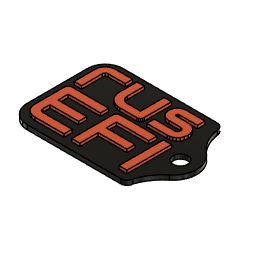
THIN - Keychain_v2 v1 (Autodesk Fusion 360 design; units mm, degrees)
Autodesk Fusion 360 part; units mm, degrees
note: some values were not read from the file. Set by a fixed rule: which sketch regions a step uses.
sketch "Sketch1" plane through (0, 0, 0) normal (0, 0, 1) x (1, 0, 0)
  line L0 (0, 0) -> (0, 17)
  line L1 (46.7294, 0) -> (46.7294, 50.0165)
  line L2 (9.2279, 24.9581) -> (3.5574, 24.9581)
  spline S0 degree 2 poles (3.5574, 24.9581) (3.0437, 24.9581) (2.7819, 24.7012) knots 0 0 0 1 1 1
  spline S1 degree 2 poles (2.7819, 24.7012) (2.5202, 24.4443) (2.5202, 23.95) knots 0 0 0 1 1 1
  line L3 (2.5202, 23.95) -> (2.5202, 17)
  line L4 (2.5202, 17) -> (0, 17)
  line L5 (0, 17) -> (0, 23.95)
  spline S2 degree 2 poles (0, 23.95) (0, 24.5994) (0.1648, 25.1132) knots 0 0 0 1 1 1
  spline S3 degree 2 poles (0.1648, 25.1132) (0.3296, 25.6269) (0.6058, 26.0195) knots 0 0 0 1 1 1
  spline S4 degree 2 poles (0.6058, 26.0195) (0.8821, 26.4121) (1.2407, 26.6883) knots 0 0 0 1 1 1
  spline S5 degree 2 poles (1.2407, 26.6883) (1.5994, 26.9646) (1.9919, 27.139) knots 0 0 0 1 1 1
  spline S6 degree 2 poles (1.9919, 27.139) (2.3845, 27.3135) (2.7868, 27.3959) knots 0 0 0 1 1 1
  spline S7 degree 2 poles (2.7868, 27.3959) (3.1891, 27.4783) (3.538, 27.4783) knots 0 0 0 1 1 1
  line L6 (3.538, 27.4783) -> (9.2279, 27.4783)
  line L7 (9.2279, 27.4783) -> (9.2279, 24.9581)
  spline S8 degree 2 poles (22.3427, 18.2698) (22.3427, 17.9984) (22.2458, 17.7658) knots 0 0 0 1 1 1
  spline S9 degree 2 poles (22.2458, 17.7658) (22.1489, 17.5331) (21.9793, 17.3635) knots 0 0 0 1 1 1
  spline S10 degree 2 poles (21.9793, 17.3635) (21.8096, 17.1939) (21.5818, 17.0969) knots 0 0 0 1 1 1
  spline S11 degree 2 poles (21.5818, 17.0969) (21.354, 17) (21.0923, 17) knots 0 0 0 1 1 1
  line L8 (21.0923, 17) -> (15.3927, 17)
  spline S12 degree 2 poles (15.3927, 17) (14.9275, 17) (14.3992, 17.1066) knots 0 0 0 1 1 1
  spline S13 degree 2 poles (14.3992, 17.1066) (13.8709, 17.2132) (13.3572, 17.4507) knots 0 0 0 1 1 1
  spline S14 degree 2 poles (13.3572, 17.4507) (12.8434, 17.6882) (12.3636, 18.0517) knots 0 0 0 1 1 1
  spline S15 degree 2 poles (12.3636, 18.0517) (11.8838, 18.4152) (11.5252, 18.9338) knots 0 0 0 1 1 1
  spline S16 degree 2 poles (11.5252, 18.9338) (11.1665, 19.4524) (10.9484, 20.1309) knots 0 0 0 1 1 1
  spline S17 degree 2 poles (10.9484, 20.1309) (10.7303, 20.8094) (10.7303, 21.6624) knots 0 0 0 1 1 1
  line L9 (10.7303, 21.6624) -> (10.7303, 27.4783)
  line L10 (10.7303, 27.4783) -> (13.2506, 27.4783)
  line L11 (13.2506, 27.4783) -> (13.2506, 21.6624)
  spline S18 degree 2 poles (13.2506, 21.6624) (13.2506, 21.1681) (13.4202, 20.7755) knots 0 0 0 1 1 1
  spline S19 degree 2 poles (13.4202, 20.7755) (13.5898, 20.3829) (13.8806, 20.1018) knots 0 0 0 1 1 1
  spline S20 degree 2 poles (13.8806, 20.1018) (14.1714, 19.8207) (14.564, 19.6705) knots 0 0 0 1 1 1
  spline S21 degree 2 poles (14.564, 19.6705) (14.9566, 19.5202) (15.4121, 19.5202) knots 0 0 0 1 1 1
  line L12 (15.4121, 19.5202) -> (19.8225, 19.5202)
  line L13 (19.8225, 19.5202) -> (19.8225, 27.4783)
  line L14 (19.8225, 27.4783) -> (22.3427, 27.4783)
  line L15 (22.3427, 27.4783) -> (22.3427, 18.2698)
  spline S22 degree 2 poles (34.8372, 20.538) (34.8372, 19.8886) (34.6725, 19.37) knots 0 0 0 1 1 1
  spline S23 degree 2 poles (34.6725, 19.37) (34.5077, 18.8514) (34.2363, 18.4588) knots 0 0 0 1 1 1
  spline S24 degree 2 poles (34.2363, 18.4588) (33.9649, 18.0662) (33.6062, 17.79) knots 0 0 0 1 1 1
  spline S25 degree 2 poles (33.6062, 17.79) (33.2476, 17.5137) (32.855, 17.3393) knots 0 0 0 1 1 1
  spline S26 degree 2 poles (32.855, 17.3393) (32.4624, 17.1648) (32.0601, 17.0824) knots 0 0 0 1 1 1
  spline S27 degree 2 poles (32.0601, 17.0824) (31.6579, 17) (31.2992, 17) knots 0 0 0 1 1 1
  line L16 (31.2992, 17) -> (24.4752, 17)
  line L17 (24.4752, 17) -> (24.4752, 19.5202)
  line L18 (24.4752, 19.5202) -> (31.2798, 19.5202)
  spline S28 degree 2 poles (31.2798, 19.5202) (31.7936, 19.5202) (32.0553, 19.7819) knots 0 0 0 1 1 1
  spline S29 degree 2 poles (32.0553, 19.7819) (32.317, 20.0437) (32.317, 20.538) knots 0 0 0 1 1 1
  spline S30 degree 2 poles (32.317, 20.538) (32.2685, 21.5461) (31.2992, 21.5461) knots 0 0 0 1 1 1
  line L19 (31.2992, 21.5461) -> (27.3929, 21.5461)
  spline S31 degree 2 poles (27.3929, 21.5461) (26.5593, 21.5461) (25.9777, 21.8369) knots 0 0 0 1 1 1
  spline S32 degree 2 poles (25.9777, 21.8369) (25.3961, 22.1277) (25.0326, 22.5639) knots 0 0 0 1 1 1
  spline S33 degree 2 poles (25.0326, 22.5639) (24.6691, 23.0001) (24.5092, 23.5041) knots 0 0 0 1 1 1
  spline S34 degree 2 poles (24.5092, 23.5041) (24.3492, 24.0082) (24.3492, 24.4443) knots 0 0 0 1 1 1
  spline S35 degree 2 poles (24.3492, 24.4443) (24.3492, 25.2877) (24.6497, 25.8644) knots 0 0 0 1 1 1
  spline S36 degree 2 poles (24.6497, 25.8644) (24.9502, 26.4411) (25.4058, 26.7998) knots 0 0 0 1 1 1
  spline S37 degree 2 poles (25.4058, 26.7998) (25.8614, 27.1584) (26.3945, 27.3184) knots 0 0 0 1 1 1
  spline S38 degree 2 poles (26.3945, 27.3184) (26.9276, 27.4783) (27.3929, 27.4783) knots 0 0 0 1 1 1
  line L20 (27.3929, 27.4783) -> (33.5868, 27.4783)
  line L21 (33.5868, 27.4783) -> (33.5868, 24.9581)
  line L22 (33.5868, 24.9581) -> (27.4123, 24.9581)
  spline S39 degree 2 poles (27.4123, 24.9581) (27.2184, 24.9581) (27.1069, 24.9145) knots 0 0 0 1 1 1
  spline S40 degree 2 poles (27.1069, 24.9145) (26.9955, 24.8708) (26.9422, 24.7981) knots 0 0 0 1 1 1
  spline S41 degree 2 poles (26.9422, 24.7981) (26.8888, 24.7255) (26.8791, 24.6431) knots 0 0 0 1 1 1
  spline S42 degree 2 poles (26.8791, 24.6431) (26.8695, 24.5607) (26.8695, 24.4831) knots 0 0 0 1 1 1
  spline S43 degree 2 poles (26.8695, 24.4831) (26.8791, 24.328) (26.9276, 24.2408) knots 0 0 0 1 1 1
  spline S44 degree 2 poles (26.9276, 24.2408) (26.9761, 24.1536) (27.0488, 24.1148) knots 0 0 0 1 1 1
  spline S45 degree 2 poles (27.0488, 24.1148) (27.1215, 24.076) (27.2136, 24.0712) knots 0 0 0 1 1 1
  spline S46 degree 2 poles (27.2136, 24.0712) (27.3056, 24.0663) (27.3929, 24.0663) knots 0 0 0 1 1 1
  line L23 (27.3929, 24.0663) -> (31.2992, 24.0663)
  spline S47 degree 2 poles (31.2992, 24.0663) (32.2685, 24.0663) (32.9471, 23.7174) knots 0 0 0 1 1 1
  spline S48 degree 2 poles (32.9471, 23.7174) (33.6256, 23.3684) (34.0424, 22.8401) knots 0 0 0 1 1 1
  spline S49 degree 2 poles (34.0424, 22.8401) (34.4592, 22.3119) (34.6482, 21.6915) knots 0 0 0 1 1 1
  spline S50 degree 2 poles (34.6482, 21.6915) (34.8372, 21.0711) (34.8372, 20.538) knots 0 0 0 1 1 1
  line L24 (12.3954, 6.1297) -> (2.7197, 6.1297)
  line L25 (2.7197, 8.8703) -> (12.3954, 8.8703)
  line L26 (12.3954, 8.8703) -> (12.3954, 6.1297)
  line L27 (13.6192, 0) -> (3.8075, 0)
  spline S51 degree 2 poles (3.8075, 0) (3.2427, 0) (2.5732, 0.1987) knots 0 0 0 1 1 1
  spline S52 degree 2 poles (2.5732, 0.1987) (1.9038, 0.3975) (1.3337, 0.8525) knots 0 0 0 1 1 1
  spline S53 degree 2 poles (1.3337, 0.8525) (0.7636, 1.3075) (0.3818, 2.0345) knots 0 0 0 1 1 1
  spline S54 degree 2 poles (0.3818, 2.0345) (0, 2.7615) (0, 3.818) knots 0 0 0 1 1 1
  line L28 (0, 3.818) -> (0, 13.6297)
  spline S55 degree 2 poles (0, 13.6297) (0, 13.9121) (0.1046, 14.1632) knots 0 0 0 1 1 1
  spline S56 degree 2 poles (0.1046, 14.1632) (0.2092, 14.4142) (0.3923, 14.6025) knots 0 0 0 1 1 1
  spline S57 degree 2 poles (0.3923, 14.6025) (0.5753, 14.7908) (0.8264, 14.8954) knots 0 0 0 1 1 1
  spline S58 degree 2 poles (0.8264, 14.8954) (1.0774, 15) (1.3703, 15) knots 0 0 0 1 1 1
  line L29 (1.3703, 15) -> (13.6192, 15)
  line L30 (13.6192, 15) -> (13.6192, 12.2803)
  line L31 (13.6192, 12.2803) -> (2.7197, 12.2803)
  spline S59 degree 2 poles (2.7197, 3.818) (2.7197, 3.2845) (3.0021, 3.0021) knots 0 0 0 1 1 1
  spline S60 degree 2 poles (3.0021, 3.0021) (3.2845, 2.7197) (3.8285, 2.7197) knots 0 0 0 1 1 1
  line L32 (3.8285, 2.7197) -> (13.6192, 2.7197)
  line L33 (13.6192, 2.7197) -> (13.6192, 0)
  line L34 (28.6506, 6.1297) -> (18.9644, 6.1297)
  line L35 (18.9644, 8.8703) -> (28.6506, 8.8703)
  line L36 (28.6506, 8.8703) -> (28.6506, 6.1297)
  line L37 (29.864, 12.2803) -> (18.9644, 12.2803)
  line L38 (18.9644, 0) -> (16.2448, 0)
  line L39 (16.2448, 0) -> (16.2448, 13.6297)
  spline S61 degree 2 poles (16.2448, 13.6297) (16.2448, 13.9121) (16.3494, 14.1632) knots 0 0 0 1 1 1
  spline S62 degree 2 poles (16.3494, 14.1632) (16.454, 14.4142) (16.637, 14.6025) knots 0 0 0 1 1 1
  spline S63 degree 2 poles (16.637, 14.6025) (16.8201, 14.7908) (17.0711, 14.8954) knots 0 0 0 1 1 1
  spline S64 degree 2 poles (17.0711, 14.8954) (17.3222, 15) (17.6151, 15) knots 0 0 0 1 1 1
  line L40 (17.6151, 15) -> (29.864, 15)
  line L41 (29.864, 15) -> (29.864, 12.2803)
  line L42 (34.8013, 0) -> (32.0816, 0)
  line L43 (32.0816, 0) -> (32.0816, 15)
  line L44 (32.0816, 15) -> (34.8013, 15)
  line L45 (34.8013, 15) -> (34.8013, 0)
  line L46 (2.7197, 12.2803) -> (2.7197, 8.8703)
  line L47 (2.7197, 6.1297) -> (2.7197, 3.818)
  line L48 (18.9644, 12.2803) -> (18.9644, 8.8703)
  line L49 (18.9644, 6.1297) -> (18.9644, 0)
  constraint coincident L24.end L46
  constraint coincident L34.end L48
  constraint collinear L46 L47
  constraint collinear L48 L49
sketch "Sketch2" plane through (0, 0, 0) normal (0, 0, 1) x (1, 0, 0)
  line L0 (3.538, 29.9783) -> (35.2726, 29.9781)
  line L1 (-2.5, 3.818) -> (-2.5, 23.95)
  spline S0 degree 3 poles (-2.5, 23.95) (-2.5, 24.5944) (-2.4192, 25.2425) (-2.2158, 25.8767) knots 0 0 0 0 1 1 1 1
  spline S1 degree 3 poles (-2.2158, 25.8767) (-2.0384, 26.4298) (-1.7836, 26.9681) (-1.4387, 27.4582) knots 0 0 0 0 1 1 1 1
  spline S2 degree 3 poles (-1.4387, 27.4582) (-1.1203, 27.9106) (-0.7316, 28.3247) (-0.2848, 28.6689) knots 0 0 0 0 1 1 1 1
  spline S3 degree 3 poles (-0.2848, 28.6689) (0.102, 28.9669) (0.5256, 29.2231) (0.9766, 29.4236) knots 0.000003 0.000003 0.000003 0.000003 1 1 1 1
  spline S4 degree 3 poles (0.9766, 29.4236) (1.3945, 29.6093) (1.8337, 29.7526) (2.2852, 29.8451) knots 0 0 0 0 1 1 1 1
  spline S5 degree 3 poles (2.2852, 29.8451) (2.6925, 29.9285) (3.1086, 29.9783) (3.538, 29.9783) knots 0.000006 0.000006 0.000006 0.000006 1 1 1 1
  line L2 (35.302, -2.5) -> (3.8075, -2.5)
  spline S6 degree 3 poles (3.8075, -2.5) (3.1378, -2.5) (2.4919, -2.385) (1.8617, -2.1979) knots 0 0 0 0 1 1 1 1
  spline S7 degree 3 poles (1.8617, -2.1979) (1.102, -1.9723) (0.3884, -1.5917) (-0.2259, -1.1014) knots 0.000003 0.000003 0.000003 0.000003 1 1 1 1
  spline S8 degree 3 poles (-0.2259, -1.1014) (-0.9006, -0.5629) (-1.4387, 0.1241) (-1.8315, 0.8721) knots 0.000002 0.000002 0.000002 0.000002 1 1 1 1
  spline S9 degree 3 poles (-1.8315, 0.8721) (-2.3179, 1.7981) (-2.5, 2.8125) (-2.5, 3.818) knots 0 0 0 0 1 1 1 1
  line L3 (37.3013, 12.981) -> (47.3013, 13.0001) construction
  circle A0 centre (41.3001, 12.886) radius 4 construction
  arc A1 (45.3013, 12.9963) -> (37.286, 20.981) centre (37.3013, 12.981) ccw
  line L4 (37.2726, 27.9819) -> (37.286, 20.981)
  line L5 (37.3013, 12.981) -> (37.3166, 4.981)
  line L6 (37.286, 20.981) -> (37.3013, 12.981)
  line L7 (37.3166, 4.981) -> (37.302, -0.5053)
  arc A2 (37.3166, 4.981) -> (45.3013, 12.9963) centre (37.3013, 12.981) ccw
  line L8 (37.2963, 15.5591) -> (37.2772, 25.5591) construction
  line L9 (37.3099, 8.4845) -> (37.329, -1.5154) construction
  arc A3 (35.302, -2.5) -> (37.302, -0.5053) centre (35.302, -0.5) ccw
  arc A4 (37.2726, 27.9819) -> (35.2726, 29.9781) centre (35.2726, 27.9781) ccw
  circle A5 centre (39.8013, 12.982) radius 2.5
  line L10 (42.3013, 12.9905) -> (42.2893, 19.2355) construction
  line L11 (42.3013, 12.9905) -> (42.3132, 6.7456) construction
  arc A6 (37.2726, 27.9819) -> (42.2893, 19.2355) centre (50.8322, 29.9474) ccw
  arc A7 (42.3132, 6.7456) -> (37.302, -0.5053) centre (52.0006, -5.3068) ccw
  dimension "d14" = 10
  dimension "d16" = 8
  dimension "d20" = 10
  dimension "d21" = 10
  dimension "d26" = 2
  dimension "d27" = 2
  dimension "d28" = 5
  constraint coincident S5 L0.start
  constraint coincident L0 S5.end
  constraint perpendicular L3 L4
  constraint coincident L3.start A0
  constraint coincident L3.start A1.centre
  constraint tangent A0 A1
  constraint coincident L5.end L4
  constraint coincident L3.start L4
  constraint coincident L3 A1.start
  constraint concentric A1 A2
  constraint coincident L6 L8.start
  constraint coincident L5 L9.start
  constraint tangent L2 A3
  constraint tangent L7 A3
  constraint tangent L0 A4
  constraint tangent L4 A4
  constraint coincident L3.start A5
  constraint midpoint L3 L10.start
  constraint coincident A1 L10.end
  constraint perpendicular L3 L10
  constraint coincident A2 L11.end
  constraint parallel L10 L11
  constraint tangent A1 A6
  constraint tangent A2 A7
  measures "d14" distance of L3.start L3.end
  measures "d16" diameter of A0
  measures "d20" distance of L8.start L8.end
  measures "d21" distance of L9.start L9.end
  measures "d26" radius of A3
  measures "d27" radius of A4
  measures "d28" diameter of A5
extrude "Extrude1" add sketch "Sketch1" along normal blind 2.5 makes body 1 at (17.1513, 6.5865, 0) makes body 2 at (1.6801, 19.3167, 0) makes body 3 at (33.8947, 5, 0) makes body 4 at (29.0181, 17.8401, 0) makes body 5 at (21.5027, 21.7561, 0) makes body 6 at (0.9066, 8.7727, 0)
extrude "Extrude2" cut sketch "Sketch2" along normal blind 1.5 contours L0 L1 S0 S1 S2 S3 S4 S5 L2 S6 S7 S8 S9 L4 L5 L6 L7 A3 A4 bodies 1 2 3 4 5 6
extrude "Extrude3" add sketch "Sketch2" along normal blind 1.5 separate body contours L0 L1 S0 S1 S2 S3 S4 S5 L2 S6 S7 S8 S9 L4 L5 L6 L7 A3 A4 makes body 7
extrude "Extrude5" add sketch "Sketch2" along normal up to surface (1.5 mm away) contours A1 L4 A6 | A1 L5 L6 A2 | L7 A2 A7 bodies 7
sketch "Sketch4" plane through (0, 0, 0) normal (0, 0, 1) x (1, 0, 0)
  line L0 (-2.5, 3.818) -> (-2.5, 23.95) construction
  line L1 (37.3013, 12.981) -> (-2.5, 12.981) construction
  spline S0 degree 2 poles (31.8619, 9.7118) (31.8619, 9.5612) (31.9205, 9.4301) knots 0 0 0 1 1 1
  spline S1 degree 2 poles (31.9205, 9.4301) (31.9791, 9.299) (32.0767, 9.2014) knots 0 0 0 1 1 1
  spline S2 degree 2 poles (32.0767, 9.2014) (32.1744, 9.1037) (32.3055, 9.0479) knots 0 0 0 1 1 1
  spline S3 degree 2 poles (32.3055, 9.0479) (32.4366, 8.9921) (32.5816, 8.9921) knots 0 0 0 1 1 1
  spline S4 degree 2 poles (32.5816, 8.9921) (32.7322, 8.9921) (32.8633, 9.0479) knots 0 0 0 1 1 1
  spline S5 degree 2 poles (32.8633, 9.0479) (32.9944, 9.1037) (33.0921, 9.2014) knots 0 0 0 1 1 1
  spline S6 degree 2 poles (33.0921, 9.2014) (33.1897, 9.299) (33.2455, 9.4301) knots 0 0 0 1 1 1
  spline S7 degree 2 poles (33.2455, 9.4301) (33.3013, 9.5612) (33.3013, 9.7118) knots 0 0 0 1 1 1
  spline S8 degree 2 poles (33.3013, 9.7118) (33.3013, 9.8569) (33.2455, 9.988) knots 0 0 0 1 1 1
  spline S9 degree 2 poles (33.2455, 9.988) (33.1897, 10.1191) (33.0921, 10.2167) knots 0 0 0 1 1 1
  spline S10 degree 2 poles (33.0921, 10.2167) (32.9944, 10.3143) (32.8633, 10.3729) knots 0 0 0 1 1 1
  spline S11 degree 2 poles (32.8633, 10.3729) (32.7322, 10.4315) (32.5816, 10.4315) knots 0 0 0 1 1 1
  spline S12 degree 2 poles (32.5816, 10.4315) (32.4366, 10.4315) (32.3055, 10.3729) knots 0 0 0 1 1 1
  spline S13 degree 2 poles (32.3055, 10.3729) (32.1744, 10.3143) (32.0767, 10.2167) knots 0 0 0 1 1 1
  spline S14 degree 2 poles (32.0767, 10.2167) (31.9791, 10.1191) (31.9205, 9.988) knots 0 0 0 1 1 1
  spline S15 degree 2 poles (31.9205, 9.988) (31.8619, 9.8569) (31.8619, 9.7118) knots 0 0 0 1 1 1
  line L2 (23.4045, 8.981) -> (28.6374, 8.981)
  spline S16 degree 2 poles (28.6374, 8.981) (28.8382, 8.981) (29.0698, 9.0284) knots 0 0 0 1 1 1
  spline S17 degree 2 poles (29.0698, 9.0284) (29.3013, 9.0758) (29.5272, 9.1762) knots 0 0 0 1 1 1
  spline S18 degree 2 poles (29.5272, 9.1762) (29.7532, 9.2767) (29.9596, 9.4357) knots 0 0 0 1 1 1
  spline S19 degree 2 poles (29.9596, 9.4357) (30.166, 9.5947) (30.325, 9.8206) knots 0 0 0 1 1 1
  spline S20 degree 2 poles (30.325, 9.8206) (30.484, 10.0465) (30.5788, 10.345) knots 0 0 0 1 1 1
  spline S21 degree 2 poles (30.5788, 10.345) (30.6737, 10.6435) (30.6737, 11.0173) knots 0 0 0 1 1 1
  line L3 (30.6737, 11.0173) -> (30.6737, 14.9447)
  spline S22 degree 2 poles (30.6737, 14.9447) (30.6737, 15.1456) (30.6262, 15.3771) knots 0 0 0 1 1 1
  spline S23 degree 2 poles (30.6262, 15.3771) (30.5788, 15.6086) (30.4784, 15.8345) knots 0 0 0 1 1 1
  spline S24 degree 2 poles (30.4784, 15.8345) (30.378, 16.0605) (30.2162, 16.2669) knots 0 0 0 1 1 1
  spline S25 degree 2 poles (30.2162, 16.2669) (30.0544, 16.4733) (29.8285, 16.6323) knots 0 0 0 1 1 1
  spline S26 degree 2 poles (29.8285, 16.6323) (29.6025, 16.7913) (29.3069, 16.8862) knots 0 0 0 1 1 1
  spline S27 degree 2 poles (29.3069, 16.8862) (29.0112, 16.981) (28.6374, 16.981) knots 0 0 0 1 1 1
  line L4 (28.6374, 16.981) -> (23.4045, 16.981)
  line L5 (23.4045, 16.981) -> (23.4045, 15.5305)
  line L6 (23.4045, 15.5305) -> (28.6374, 15.5305)
  spline S28 degree 2 poles (28.6374, 15.5305) (28.9219, 15.5305) (29.0725, 15.3799) knots 0 0 0 1 1 1
  spline S29 degree 2 poles (29.0725, 15.3799) (29.2232, 15.2292) (29.2232, 14.9336) knots 0 0 0 1 1 1
  line L7 (29.2232, 14.9336) -> (29.2232, 11.0173)
  spline S30 degree 2 poles (29.2232, 11.0173) (29.2232, 10.7383) (29.0698, 10.5849) knots 0 0 0 1 1 1
  spline S31 degree 2 poles (29.0698, 10.5849) (28.9163, 10.4315) (28.6374, 10.4315) knots 0 0 0 1 1 1
  line L8 (28.6374, 10.4315) -> (23.4045, 10.4315)
  line L9 (23.4045, 10.4315) -> (23.4045, 8.981)
  spline S32 degree 2 poles (13.636, 12.2167) (13.636, 11.4859) (13.887, 10.8722) knots 0 0 0 1 1 1
  spline S33 degree 2 poles (13.887, 10.8722) (14.1381, 10.2585) (14.5844, 9.8122) knots 0 0 0 1 1 1
  spline S34 degree 2 poles (14.5844, 9.8122) (15.0307, 9.3659) (15.6416, 9.1177) knots 0 0 0 1 1 1
  spline S35 degree 2 poles (15.6416, 9.1177) (16.2525, 8.8694) (16.9721, 8.8694) knots 0 0 0 1 1 1
  line L10 (16.9721, 8.8694) -> (18.9359, 8.8694)
  spline S36 degree 2 poles (18.9359, 8.8694) (19.6555, 8.8694) (20.2692, 9.1177) knots 0 0 0 1 1 1
  spline S37 degree 2 poles (20.2692, 9.1177) (20.8829, 9.3659) (21.3292, 9.8122) knots 0 0 0 1 1 1
  spline S38 degree 2 poles (21.3292, 9.8122) (21.7755, 10.2585) (22.0293, 10.8722) knots 0 0 0 1 1 1
  spline S39 degree 2 poles (22.0293, 10.8722) (22.2831, 11.4859) (22.2831, 12.2167) knots 0 0 0 1 1 1
  line L11 (22.2831, 12.2167) -> (22.2831, 13.7453)
  spline S40 degree 2 poles (22.2831, 13.7453) (22.2831, 14.4705) (22.0293, 15.087) knots 0 0 0 1 1 1
  spline S41 degree 2 poles (22.0293, 15.087) (21.7755, 15.7034) (21.3292, 16.147) knots 0 0 0 1 1 1
  spline S42 degree 2 poles (21.3292, 16.147) (20.8829, 16.5905) (20.2692, 16.8415) knots 0 0 0 1 1 1
  spline S43 degree 2 poles (20.2692, 16.8415) (19.6555, 17.0926) (18.9359, 17.0926) knots 0 0 0 1 1 1
  line L12 (18.9359, 17.0926) -> (16.9721, 17.0926)
  spline S44 degree 2 poles (16.9721, 17.0926) (16.2525, 17.0926) (15.6416, 16.8415) knots 0 0 0 1 1 1
  spline S45 degree 2 poles (15.6416, 16.8415) (15.0307, 16.5905) (14.5844, 16.147) knots 0 0 0 1 1 1
  spline S46 degree 2 poles (14.5844, 16.147) (14.1381, 15.7034) (13.887, 15.087) knots 0 0 0 1 1 1
  spline S47 degree 2 poles (13.887, 15.087) (13.636, 14.4705) (13.636, 13.7453) knots 0 0 0 1 1 1
  line L13 (13.636, 13.7453) -> (13.636, 12.2167)
  spline S48 degree 2 poles (15.0865, 13.7453) (15.0865, 14.1749) (15.2232, 14.5235) knots 0 0 0 1 1 1
  spline S49 degree 2 poles (15.2232, 14.5235) (15.3598, 14.8722) (15.6081, 15.1205) knots 0 0 0 1 1 1
  spline S50 degree 2 poles (15.6081, 15.1205) (15.8564, 15.3687) (16.205, 15.5054) knots 0 0 0 1 1 1
  spline S51 degree 2 poles (16.205, 15.5054) (16.5537, 15.6421) (16.9721, 15.6421) knots 0 0 0 1 1 1
  line L14 (16.9721, 15.6421) -> (18.9359, 15.6421)
  spline S52 degree 2 poles (18.9359, 15.6421) (19.3598, 15.6421) (19.7085, 15.5054) knots 0 0 0 1 1 1
  spline S53 degree 2 poles (19.7085, 15.5054) (20.0572, 15.3687) (20.3082, 15.1205) knots 0 0 0 1 1 1
  spline S54 degree 2 poles (20.3082, 15.1205) (20.5593, 14.8722) (20.696, 14.5235) knots 0 0 0 1 1 1
  spline S55 degree 2 poles (20.696, 14.5235) (20.8327, 14.1749) (20.8327, 13.7453) knots 0 0 0 1 1 1
  line L15 (20.8327, 13.7453) -> (20.8327, 12.2167)
  spline S56 degree 2 poles (20.8327, 12.2167) (20.8327, 11.7871) (20.696, 11.4385) knots 0 0 0 1 1 1
  spline S57 degree 2 poles (20.696, 11.4385) (20.5593, 11.0898) (20.3082, 10.8415) knots 0 0 0 1 1 1
  spline S58 degree 2 poles (20.3082, 10.8415) (20.0572, 10.5933) (19.7085, 10.4566) knots 0 0 0 1 1 1
  spline S59 degree 2 poles (19.7085, 10.4566) (19.3598, 10.3199) (18.9359, 10.3199) knots 0 0 0 1 1 1
  line L16 (18.9359, 10.3199) -> (16.9833, 10.3199)
  spline S60 degree 2 poles (16.9833, 10.3199) (16.5593, 10.3199) (16.2106, 10.4566) knots 0 0 0 1 1 1
  spline S61 degree 2 poles (16.2106, 10.4566) (15.8619, 10.5933) (15.6109, 10.8415) knots 0 0 0 1 1 1
  spline S62 degree 2 poles (15.6109, 10.8415) (15.3598, 11.0898) (15.2232, 11.4385) knots 0 0 0 1 1 1
  spline S63 degree 2 poles (15.2232, 11.4385) (15.0865, 11.7871) (15.0865, 12.2167) knots 0 0 0 1 1 1
  line L17 (15.0865, 12.2167) -> (15.0865, 13.7453)
  line L18 (2.8912, 8.981) -> (4.3529, 8.981)
  line L19 (4.3529, 8.981) -> (4.3529, 13.7453)
  line L20 (4.3529, 13.7453) -> (6.9247, 9.2209)
  spline S64 degree 2 poles (6.9247, 9.2209) (7.0195, 9.0479) (7.1897, 8.9587) knots 0 0 0 1 1 1
  spline S65 degree 2 poles (7.1897, 8.9587) (7.3598, 8.8694) (7.5551, 8.8694) knots 0 0 0 1 1 1
  spline S66 degree 2 poles (7.5551, 8.8694) (7.7448, 8.8694) (7.9094, 8.9587) knots 0 0 0 1 1 1
  spline S67 degree 2 poles (7.9094, 8.9587) (8.0739, 9.0479) (8.1688, 9.2209) knots 0 0 0 1 1 1
  line L21 (8.1688, 9.2209) -> (10.7518, 13.7453)
  line L22 (10.7518, 13.7453) -> (10.7518, 8.981)
  line L23 (10.7518, 8.981) -> (12.2022, 8.981)
  line L24 (12.2022, 8.981) -> (12.2022, 16.3617)
  spline S68 degree 2 poles (12.2022, 16.3617) (12.2022, 16.6128) (12.0544, 16.808) knots 0 0 0 1 1 1
  spline S69 degree 2 poles (12.0544, 16.808) (11.9066, 17.0033) (11.6667, 17.0703) knots 0 0 0 1 1 1
  spline S70 degree 2 poles (11.6667, 17.0703) (11.5495, 17.0981) (11.4324, 17.0898) knots 0 0 0 1 1 1
  spline S71 degree 2 poles (11.4324, 17.0898) (11.3152, 17.0814) (11.2064, 17.0396) knots 0 0 0 1 1 1
  spline S72 degree 2 poles (11.2064, 17.0396) (11.0976, 16.9977) (11.0084, 16.9224) knots 0 0 0 1 1 1
  spline S73 degree 2 poles (11.0084, 16.9224) (10.9191, 16.8471) (10.8578, 16.7411) knots 0 0 0 1 1 1
  line L25 (10.8578, 16.7411) -> (7.5551, 11.0005)
  line L26 (7.5551, 11.0005) -> (4.2525, 16.7411)
  spline S74 degree 2 poles (4.2525, 16.7411) (4.1241, 16.9531) (3.8982, 17.0424) knots 0 0 0 1 1 1
  spline S75 degree 2 poles (3.8982, 17.0424) (3.6723, 17.1316) (3.4268, 17.0703) knots 0 0 0 1 1 1
  spline S76 degree 2 poles (3.4268, 17.0703) (3.1925, 17.0033) (3.0419, 16.808) knots 0 0 0 1 1 1
  spline S77 degree 2 poles (3.0419, 16.808) (2.8912, 16.6128) (2.8912, 16.3617) knots 0 0 0 1 1 1
  line L27 (2.8912, 16.3617) -> (2.8912, 8.981)
  point P0 (37.3013, 12.981)
  point P1 (37.3013, 12.981)
  constraint coincident P0 L1.start
  constraint coincident L0 L1.end
  constraint perpendicular L0 L1
extrude "Extrude6" cut sketch "Sketch4" along normal blind 0.5 bodies 7
